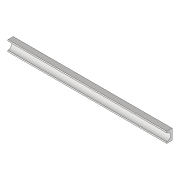
# Autodesk Inventor part: Gerade_1
Saved by Autodesk Inventor 2020 (Build 240168000, 168)
## iProperties
Created: 2020-04-19
Part Number: Gerade_1
Material: Generisch
Document SubType Name: Modeling
Designer: franz
Density: 1 g/cm^3
Appearance: Vorgabe
Author: franz
Autodesk Inventor part; units mm, degrees
ref_plane "YZ Plane" through (0, 0, 0) normal (1, 0, 0) x (0, 1, 0)
ref_plane "XZ Plane" through (0, 0, 0) normal (0, 1, 0) x (-1, 0, 0)
ref_plane "XY Plane" through (0, 0, 0) normal (0, 0, 1) x (1, 0, 0)
sketch "Skizze1" plane through (0, 0, 0) normal (1, 0, 0) x (0, 1, 0)
  arc A0 (-7.5, 0) -> (7.5, 0) centre (0, 0) ccw
  line L0 (-7.5, 0) -> (-10, 0)
  line L1 (-10, 0) -> (-10, -10)
  line L2 (-10, -10) -> (10, -10)
  line L3 (10, -10) -> (10, 0)
  line L4 (0, -12) -> (0, 2) projected
  line L5 (7.5, 0) -> (10, 0)
  line L6 (-14, 0) -> (14, 0) projected
  dimension "d0" = 20
  dimension "d1" = 7.5
  dimension "d2" = 10
  constraints: 10 end point, 3 perpendicular, 2 collinear, 2 point on circle, 1 centre point, 1 coincident, 1 horizontal, 1 point on line, 1 other
  measures "d0" distance between parallel lines of L3 L1
  measures "d1" radius of A0
  measures "d2" distance between parallel lines of L0 L2
extrude "Extrusion1" add sketch "Skizze1" along normal blind 300 contours A0 L4 L2 L1 L0 | A0 L5 L3 L2 L4
